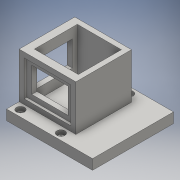
# Autodesk Inventor part: sampleChamber_test
Saved by Autodesk Inventor 2016 (Build 200138000, 138)
## iProperties
Created: 2016-04-10
Part Number: sampleChamber_test
Material: Generic
Document SubType Name: Modeling
Designer: sims01
Density: 1 g/cm^3
Appearance: Default
Author: sims01
Autodesk Inventor part; units mm, degrees
ref_plane "YZ Plane" through (0, 0, 0) normal (1, 0, 0) x (0, 1, 0)
ref_plane "XZ Plane" through (0, 0, 0) normal (0, 1, 0) x (-1, 0, 0)
ref_plane "XY Plane" through (0, 0, 0) normal (0, 0, 1) x (1, 0, 0)
sketch "Sketch1" plane through (0, 0, 0) normal (0, 0, 1) x (1, 0, 0)
  line L0 (-42.5, 40) -> (42.5, 40)
  line L1 (42.5, 40) -> (42.5, -40)
  line L2 (42.5, -40) -> (-42.5, -40)
  line L3 (-42.5, -40) -> (-42.5, 40)
  point P0 (0, 0)
  dimension "d0" = 85
  dimension "d1" = 42.5
  dimension "d2" = 80
  dimension "d3" = 40
  constraints: 8 end point, 2 parallel, 1 horizontal, 1 perpendicular
  measures "d0" distance of L1.end L2.end
  measures "d1" distance from line of point (0, 0) L1
  measures "d2" distance of L2.end L0.start
  measures "d3" distance from line of point (0, 0) L0
extrude "Extrusion1" add sketch "Sketch1" along normal blind 10
sketch "Sketch2" plane through (0, 0, 10) normal (0, 0, 1) x (1, 0, 0)
  line L0 (-42.5, 40) -> (-42.5, -40) projected
  point P0 (0, 0)
  point P1 (-35, -33.75)
  point P2 (5, -33.75)
  point P3 (-35, 33.75)
  point P4 (5, 33.75)
  dimension "d6" = 40
  dimension "d7" = 67.5
  dimension "d8" = 33.75
  dimension "d9" = 7.5
  constraints: 2 horizontal alignment, 2 vertical alignment
  measures "d6" distance of point (-35, 33.75) point (5, 33.75)
  measures "d7" distance of point (5, -33.75) point (5, 33.75)
  measures "d8" vertical distance of point (0, 0) point (5, 33.75)
  measures "d9" distance from line of L0 point (-35, 33.75)
hole "Hole1" at (-35, -33.75, 10) at (5, -33.75, 10) at (-35, 33.75, 10) at (5, 33.75, 10) direction (0, 0, -1) diameter 4.5 end through all counterbore diameter 8 counterbore depth 4 clearance for "Hex Head Cap Screw ISO 24017" size "M4" standard "ISO"
sketch "Sketch3" plane through (0, 0, 10) normal (0, 0, 1) x (1, 0, 0)
  line L0 (-42.5, 27.5) -> (13.5, 27.5)
  line L1 (13.5, 27.5) -> (13.5, -27.5)
  line L2 (13.5, -27.5) -> (-42.5, -27.5)
  line L3 (-42.5, -27.5) -> (-42.5, 27.5)
  line L4 (-42.5, 40) -> (-42.5, -40) projected
  line L5 (-35, 22.5) -> (8.5, 22.5)
  line L6 (8.5, 22.5) -> (8.5, -20)
  line L7 (8.5, -20) -> (-35, -20)
  line L8 (-35, -20) -> (-35, 22.5)
  point P0 (0, 0)
  dimension "d17" = 56
  dimension "d18" = 55
  dimension "d19" = 27.5
  dimension "d20" = 5
  dimension "d21" = 5
  dimension "d22" = 7.5
  dimension "d23" = 7.5
  constraints: 16 end point, 4 parallel, 2 horizontal, 2 perpendicular, 1 collinear
  measures "d17" distance of L0.start L0.end
  measures "d18" distance of L0.end L1.end
  measures "d19" distance from line of L2 point (0, 0)
  measures "d20" distance between parallel lines of L5 L0
  measures "d21" distance between parallel lines of L1 L6
  measures "d22" distance between parallel lines of L2 L7
  measures "d23" distance between parallel lines of L3 L8
extrude "Extrusion2" add sketch "Sketch3" along normal blind 45
sketch "Sketch4" plane through (-42.5, -27.5, 10) normal (0, -1, 0) x (1, 0, 0)
  line L0 (5, 40) -> (51, 40)
  line L1 (51, 40) -> (51, 5)
  line L2 (51, 5) -> (5, 5)
  line L3 (5, 5) -> (5, 40)
  line L4 (0, 0) -> (0, 45) projected
  line L5 (56, 0) -> (56, 45) projected
  line L6 (51, 45) -> (7.5, 45) projected
  line L7 (0, 0) -> (85, 0) projected
  point P0 (42.5, -10)
  dimension "d27" = 5
  dimension "d28" = 5
  dimension "d29" = 5
  dimension "d30" = 5
  constraints: 8 end point, 2 parallel, 1 horizontal, 1 perpendicular
  measures "d27" distance between parallel lines of L4 L3
  measures "d28" distance between parallel lines of L5 L1
  measures "d29" distance between parallel lines of L6 L0
  measures "d30" distance between parallel lines of L7 L2
extrude "Extrusion3" cut sketch "Sketch4" against normal blind 2.5
sketch "Sketch5" plane through (-42.5, -25, 10) normal (0, -1, 0) x (1, 0, 0)
  line L0 (10, 35) -> (46, 35)
  line L1 (46, 35) -> (46, 10)
  line L2 (46, 10) -> (10, 10)
  line L3 (10, 10) -> (10, 35)
  line L4 (5, 40) -> (51, 40) projected
  line L5 (5, 5) -> (5, 40) projected
  line L6 (51, 5) -> (5, 5) projected
  line L7 (51, 40) -> (51, 5) projected
  point P0 (42.5, -10)
  dimension "d33" = 5
  dimension "d34" = 5
  dimension "d35" = 5
  dimension "d36" = 5
  constraints: 8 end point, 2 parallel, 1 horizontal, 1 perpendicular
  measures "d33" distance between parallel lines of L4 L0
  measures "d34" distance between parallel lines of L5 L3
  measures "d35" distance between parallel lines of L6 L2
  measures "d36" distance between parallel lines of L7 L1
extrude "Extrusion4" cut sketch "Sketch5" against normal up to surface (5 mm away) contours L0 L1 L2 L3
sketch "Sketch6" plane through (-42.5, -40, 0) normal (-1, 0, 0) x (0, 0, 1)
  line L0 (50, 62.5) -> (15, 62.5)
  line L1 (15, 62.5) -> (15, 17.5)
  line L2 (15, 17.5) -> (50, 17.5)
  line L3 (50, 17.5) -> (50, 62.5)
  line L4 (55, 67.5) -> (55, 12.5) projected
  line L5 (10, 67.5) -> (55, 67.5) projected
  line L6 (10, 80) -> (10, 67.5) projected
  line L7 (10, 12.5) -> (55, 12.5) projected
  point P0 (0, 40)
  dimension "d39" = 5
  dimension "d40" = 5
  dimension "d41" = 5
  dimension "d42" = 5
  constraints: 8 end point, 2 parallel, 1 horizontal, 1 perpendicular
  measures "d39" distance between parallel lines of L4 L3
  measures "d40" distance between parallel lines of L5 L0
  measures "d41" distance between parallel lines of L6 L1
  measures "d42" distance between parallel lines of L7 L2
extrude "Extrusion5" cut sketch "Sketch6" against normal blind 2.5
sketch "Sketch7" plane through (-40, -40, 0) normal (-1, 0, 0) x (0, 0, 1)
  line L0 (45, 57.5) -> (20, 57.5)
  line L1 (20, 57.5) -> (20, 22.5)
  line L2 (20, 22.5) -> (45, 22.5)
  line L3 (45, 22.5) -> (45, 57.5)
  line L4 (50, 62.5) -> (50, 17.5) projected
  line L5 (50, 17.5) -> (15, 17.5) projected
  line L6 (15, 17.5) -> (15, 62.5) projected
  line L7 (15, 62.5) -> (50, 62.5) projected
  point P0 (0, 40)
  dimension "d45" = 5
  dimension "d46" = 5
  dimension "d47" = 5
  dimension "d48" = 5
  constraints: 8 end point, 2 parallel, 1 horizontal, 1 perpendicular
  measures "d45" distance between parallel lines of L3 L4
  measures "d46" distance between parallel lines of L5 L2
  measures "d47" distance between parallel lines of L6 L1
  measures "d48" distance between parallel lines of L7 L0
extrude "Extrusion6" cut sketch "Sketch7" against normal up to surface (5 mm away) contours L3 L2 L1 L0
equation "\"d1\" = 0.5 * d0"
equation "\"d3\" = 0.5 * d2"
equation "\"d8\" = 0.5 * d7"
equation "\"d19\" = 0.5 * d18"
equation "\"d21\" = d20"
body "Solid1"
